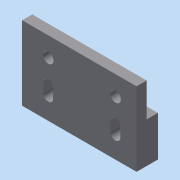
# Autodesk Inventor part: cellSTORM_Alvium_cameraadapter
Saved by Autodesk Inventor 2019.4 (Build 234330000, 330)
## iProperties
Created: 2020-12-02
Part Number: cellSTORM_Alvium_cameraadapter
Material: Generic
Document SubType Name: Modeling
Designer: diederichbenedict
Density: 1 g/cm^3
Appearance: Default
Author: diederichbenedict
Autodesk Inventor part; units mm, degrees
ref_plane "YZ Plane" through (0, 0, 0) normal (1, 0, 0) x (0, 1, 0)
ref_plane "XZ Plane" through (0, 0, 0) normal (0, 1, 0) x (-1, 0, 0)
ref_plane "Work Plane1" through (0, 0, 0) normal (0, 0, 1) x (1, 0, 0)
sketch "Sketch1" plane through (0, 0, 0) normal (0, 0, 1) x (1, 0, 0)
  circle A0 centre (-24.675, -5.1) radius 1.25 projected
  circle A1 centre (-4.675, -5.1) radius 1.25 projected
  line L0 (-32.4114, -2.1) -> (22.9321, -2.1) construction
  line L1 (-32.4114, -2.4674) -> (1.5886, -2.4674)
  line L2 (1.5886, -2.4674) -> (1.5886, -14.4674)
  line L3 (1.5886, -14.4674) -> (-32.4114, -14.4674)
  line L4 (-32.4114, -14.4674) -> (-32.4114, -2.4674)
  circle A2 centre (-24.675, -5.1) radius 1.45
  circle A3 centre (-4.675, -5.1) radius 1.45
  line L5 (-24.675, -5.1) -> (-24.675, -8.1)
  line L6 (-23.225, -5.1) -> (-23.225, -8.1)
  line L7 (-26.125, -8.1) -> (-26.125, -5.1)
  arc A4 (-23.225, -5.1) -> (-26.125, -5.1) centre (-24.675, -5.1) ccw
  arc A5 (-26.125, -8.1) -> (-23.225, -8.1) centre (-24.675, -8.1) ccw
  line L8 (-4.675, -5.1) -> (-4.675, -8.1)
  line L9 (-6.125, -5.1) -> (-6.125, -8.1)
  line L10 (-3.225, -8.1) -> (-3.225, -5.1)
  arc A6 (-3.225, -5.1) -> (-6.125, -5.1) centre (-4.675, -5.1) ccw
  arc A7 (-6.125, -8.1) -> (-3.225, -8.1) centre (-4.675, -8.1) ccw
  point P0 (0, 0)
  point P1 (-24.675, -6.6)
  point P2 (-4.675, -6.6)
  dimension "d0" = 34
  dimension "d1" = 12
  dimension "d2" = 2.9
  dimension "d3" = 2.9
  dimension "d4" = 3
  dimension "d5" = 3
  constraints: 24 end point, 8 point on circle, 8 tangent, 6 centre point, 4 parallel, 2 coincident, 2 concentric, 2 midpoint, 2 vertical, 1 horizontal, 1 perpendicular
  measures "d0" distance of L2.end L3.end
  measures "d1" distance of L1.end L2.end
  measures "d2" diameter of A2
  measures "d3" diameter of A3
  measures "d4" distance of L5.start L5.end
  measures "d5" distance of L8.start L8.end
ref_plane "Work Plane2" through (-108.8568, -31.2741, 3.325) normal (0, 0, 1) x (0.8192, 0.5736, 0)
extrude "Extrusion1" add sketch "Sketch1" along normal up to surface (3.325 mm away) contours L1 L2 L3 L4
sketch "Sketch2" plane through (-32.4114, -2.4674, 3.325) normal (0, 0, 1) x (1, 0, 0)
  circle A0 centre (27.7364, 4.2761) radius 1.6 projected
  circle A1 centre (7.7364, 4.2761) radius 1.6 projected
  line L0 (-8.2471, 157.2957) -> (-14.2937, 153.0618) projected
  line L1 (8.339, 104.3183) -> (-14.2937, 153.0618) projected
  line L2 (8.339, 104.3183) -> (0.8847, 99.0987) projected
  line L3 (0.8847, 99.0987) -> (0, 100.3623) projected
  line L4 (0, 100.3623) -> (0, 0.3674) projected
  line L5 (0, 0.3674) -> (55.3435, 0.3674) projected
  line L6 (55.3435, 0.3674) -> (57.5639, -2.8038) projected
  line L7 (57.5639, -2.8038) -> (65.7554, 2.932) projected
  line L8 (65.7554, 2.932) -> (31.3409, 52.0811) projected
  line L9 (31.3409, 52.0811) -> (41.1707, 58.964) projected
  line L10 (41.1707, 58.964) -> (36.2423, 66.0024) projected
  arc A2 (34.9764, 70.0175) -> (36.2423, 66.0024) centre (41.9764, 70.0175) ccw projected
  line L11 (34.9764, 70.0175) -> (34.9764, 131.4195) projected
  arc A3 (34.9764, 131.4195) -> (31.2086, 137.6285) centre (27.9764, 131.4195) ccw projected
  line L12 (31.2086, 137.6285) -> (10.9451, 148.1771) projected
  arc A4 (10.9451, 148.1771) -> (3.6978, 147.7021) centre (7.7129, 141.968) ccw projected
  line L13 (3.6978, 147.7021) -> (0.1902, 145.246) projected
  line L14 (-8.2471, 157.2957) -> (0.1902, 145.246) projected
  line L15 (6.7364, -8.3116) -> (6.7364, -9.6116) projected
  line L16 (7.7364, -12.1836) -> (7.7364, -9.6116) projected
  line L17 (34, 0) -> (34, -12) projected
  line L18 (0, 0) -> (34, 0) projected
  line L19 (0, -12) -> (0, 0) projected
  line L20 (34, -12) -> (0, -12) projected
  arc A5 (6.2864, -5.6326) -> (9.1864, -5.6326) centre (7.7364, -5.6326) ccw projected
  line L21 (6.2864, -2.6326) -> (6.2864, -5.6326) projected
  arc A6 (9.1864, -2.6326) -> (6.2864, -2.6326) centre (7.7364, -2.6326) ccw projected
  line L22 (9.1864, -5.6326) -> (9.1864, -2.6326) projected
  arc A7 (29.1864, -2.6326) -> (26.2864, -2.6326) centre (27.7364, -2.6326) ccw projected
  line L23 (29.1864, -5.6326) -> (29.1864, -2.6326) projected
  arc A8 (26.2864, -5.6326) -> (29.1864, -5.6326) centre (27.7364, -5.6326) ccw projected
  line L24 (26.2864, -2.6326) -> (26.2864, -5.6326) projected
  line L25 (0, 0) -> (34, 0) projected
  line L26 (0, 0) -> (34, 0)
  line L27 (34, 0) -> (34, 10)
  line L28 (34, 10) -> (0, 10)
  line L29 (0, 10) -> (0, 0)
  point P0 (32.4114, 2.4674)
  dimension "d8" = 10
  constraints: 8 end point, 2 parallel, 1 horizontal, 1 perpendicular
  measures "d8" distance of L27.end L26.end
extrude "Extrusion2" add sketch "Sketch2" along normal blind 3 contours L28 L27 L5 L4 | L5 L27 L18 L29 | L18 L17 L20 L19
body "Solid1"
